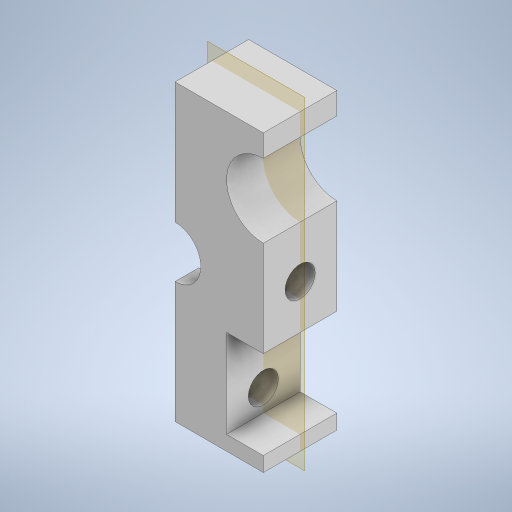
# Autodesk Inventor part: POMSliderMotor
Saved by Autodesk Inventor 2023 (Build 270158000, 158)
## iProperties
Created: 2023-03-27
Part Number: POMSliderMotor
Material: Generic
Document SubType Name: Modeling
Designer: Nathann
Density: 1 g/cm^3
Appearance: Default
Author: Nathann
Autodesk Inventor part; units mm, degrees
ref_plane "YZ Plane" through (0, 0, 0) normal (1, 0, 0) x (0, 1, 0)
ref_plane "XZ Plane" through (0, 0, 0) normal (0, 1, 0) x (-1, 0, 0)
ref_plane "XY Plane" through (0, 0, 0) normal (0, 0, 1) x (1, 0, 0)
sketch "Sketch1" plane through (0, 0, 0) normal (0, 0, 1) x (1, 0, 0)
  line L0 (10, -10) -> (-10, -10)
  line L1 (-10, -10) -> (-10, 10)
  line L2 (-10, 10) -> (10, 10)
  line L3 (10, 10) -> (10, -10)
  line L4 (10, -10) -> (-10, 10) construction
  line L5 (-10, -10) -> (10, 10) construction
  line L6 (10, -10) -> (6, -10)
  line L7 (6, -10) -> (6, 10)
  line L8 (6, 10) -> (10, 10)
  line L9 (10, 10) -> (10, -10)
  line L10 (6, 2) -> (4, 2)
  line L11 (4, 2) -> (4, -2)
  line L12 (4, -2) -> (6, -2)
  line L13 (6, -2) -> (6, 2)
  line L14 (0, 10) -> (0, -10)
  point P0 (0, 0)
  dimension "d0" = 20
  dimension "d1" = 20
  dimension "d2" = 4
  dimension "d6" = 2
  dimension "d7" = 2
  dimension "d8" = 4
  dimension "d9" = 2
  dimension "d44" = 6
  constraints: 30 end point, 6 parallel, 4 midpoint, 3 horizontal, 3 perpendicular, 3 point on line
  measures "d0" distance of L1.end L2.end
  measures "d1" distance of L0.end L1.end
  measures "d2" distance between parallel lines of L3 L7
  measures "d6" distance from line of L10 point (0, 0)
  measures "d7" distance from line of L12 point (0, 0)
  measures "d8" distance of L10.end L11.end
  measures "d9" distance of L10.start L10.end
  measures "d44" distance between parallel lines of L7 L14
extrude "Extrusion1" add sketch "Sketch1" along normal blind 5 contours L0 L14 L2 L7 L10 L11 L12
ref_plane "Work Plane1" through (0, 0, 2.5) normal (0, 0, 1) x (1, 0, 0)
sketch "Sketch2" plane through (0, 0, 2.5) normal (0, 0, 1) x (1, 0, 0)
  line L0 (0, 10) -> (0, -10) projected
  line L1 (0, 2.8868) -> (2.5, 1.4434)
  line L2 (2.5, 1.4434) -> (2.5, -1.4434)
  line L3 (2.5, -1.4434) -> (0, -2.8868)
  line L4 (0, -2.8868) -> (-2.5, -1.4434)
  line L5 (-2.5, -1.4434) -> (-2.5, 1.4434)
  line L6 (-2.5, 1.4434) -> (0, 2.8868)
  point P0 (0, 0)
  point P1 (0, 0)
  dimension "d12" = 5
  constraints: 12 end point, 1 coincident, 1 point on line, 13 other
  measures "d12" distance between parallel lines of L2 L5
extrude "Extrusion2" cut sketch "Sketch2" along normal mid plane 1.8
sketch "Sketch3" plane through (0, 0, 5) normal (0, 0, 1) x (1, 0, 0)
  circle A0 centre (0, 0) radius 1.75
  dimension "d15" = 3.5
  constraints: 1 centre point, 1 coincident
  measures "d15" diameter of A0
extrude "Extrusion3" cut sketch "Sketch3" against normal blind 8
sketch "Sketch4" plane through (0, 10, 0) normal (-1, 0, 0) x (0, 0, 1)
  circle A0 centre (2.5, -2.5) radius 1.025
  circle A1 centre (2.5, -17.5) radius 1.025
  line L0 (0, 0) -> (5, 0) projected
  line L1 (0, 0) -> (0, -8.25) projected
  line L2 (0, -11.75) -> (0, -20) projected
  line L3 (0, -20) -> (5, -20) projected
  point P0 (0, -10)
  dimension "d18" = 2.05
  dimension "d19" = 2.05
  dimension "d20" = 2.5
  dimension "d21" = 2.5
  dimension "d22" = 2.5
  dimension "d23" = 2.5
  constraints: 2 centre point
  measures "d18" diameter of A0
  measures "d19" diameter of A1
  measures "d20" distance from line of L0 A0.centre
  measures "d21" distance from line of L1 A0.centre
  measures "d22" distance from line of L2 A1.centre
  measures "d23" distance from line of L3 A1.centre
extrude "Extrusion4" cut sketch "Sketch4" against normal blind 5
sketch "Sketch5" plane through (0, 0, 0) normal (0, 0, -1) x (-1, 0, 0)
  line L0 (-4, -2) -> (-4, 2) projected
  line L1 (-6, -10) -> (-6, -2) projected
  line L2 (-4, 2) -> (-6, 2)
  line L3 (-6, 2) -> (-6, -2)
  line L4 (-6, -2) -> (-4, -2)
  line L5 (-4, -2) -> (-4, 2)
  point P0 (0, 0)
  constraints: 8 end point, 2 parallel, 1 horizontal, 1 perpendicular
extrude "Extrusion5" add sketch "Sketch5" against normal blind 5
sketch "Sketch6" plane through (0, 0, 0) normal (0, 0, -1) x (-1, 0, 0)
  line L0 (-6, -10) -> (-6, 10) projected
  circle A0 centre (-6, 6) radius 2.5
  line L1 (-6, -9) -> (-3.5, -9)
  line L2 (-3.5, -9) -> (-3.5, -3)
  line L3 (-3.5, -3) -> (-6, -3)
  line L4 (-6, -3) -> (-6, -9)
  line L5 (0, -10) -> (-6, -10) projected
  line L6 (-6, 10) -> (0, 10) projected
  point P0 (0, 0)
  point P1 (-6, 8.5)
  point P2 (-6, 3.5)
  dimension "d32" = 2.5
  dimension "d33" = 1
  dimension "d34" = 6
  dimension "d35" = 5
  dimension "d36" = 4
  constraints: 8 end point, 2 parallel, 2 point on line, 1 centre point, 1 horizontal, 1 perpendicular
  measures "d32" distance between parallel lines of L0 L2
  measures "d33" distance between parallel lines of L5 L1
  measures "d34" distance of L1.end L2.end
  measures "d35" diameter of A0
  measures "d36" distance from line of L6 A0.centre
extrude "Extrusion6" cut sketch "Sketch6" against normal blind 5 contours L0 L3 L2 L1 | L0 A0 picked at (-5.3485, 6.5196)
sketch "Sketch7" plane through (6, -3, 0) normal (1, 0, 0) x (0, 0, -1)
  circle A0 centre (-2.5, 3) radius 1.025
  line L0 (-5, 0) -> (-5, 6.5) projected
  line L1 (0, -7) -> (-5, -7) projected
  point P0 (0, 3)
  dimension "d39" = 2.5
  dimension "d40" = 10
  dimension "d41" = 2.05
  constraints: 1 centre point
  measures "d39" distance from line of L0 A0.centre
  measures "d40" distance from line of L1 A0.centre
  measures "d41" diameter of A0
extrude "Extrusion7" cut sketch "Sketch7" against normal blind 12
equation "\"d18\" = d19"
body "Solid1"
